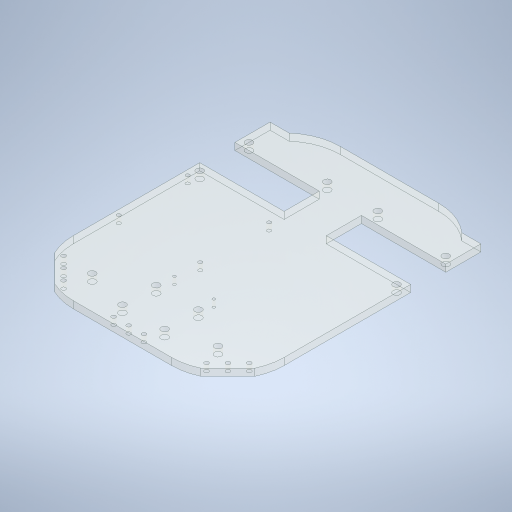
# Autodesk Inventor part: BaseP
Saved by Autodesk Inventor 2024 (Build 280153020, 153B)
## iProperties
Created: 2023-05-25
Part Number: BaseP
Material: Genérico
Document SubType Name: Modeling
Designer: victo
Density: 1 g/cm^3
Appearance: Transparente
Author: victo
Autodesk Inventor part; units mm, degrees
ref_plane "YZ Plane" through (0, 0, 0) normal (1, 0, 0) x (0, 1, 0)
ref_plane "XZ Plane" through (0, 0, 0) normal (0, 1, 0) x (-1, 0, 0)
ref_plane "XY Plane" through (0, 0, 0) normal (0, 0, 1) x (1, 0, 0)
sketch "Esboço1" plane through (0, 0, 0) normal (0, 1, 0) x (-1, 0, 0)
  line L0 (0, 0) -> (0, -190)
  line L1 (0, -190) -> (150, -190)
  line L2 (150, -190) -> (150, 0)
  line L3 (150, 0) -> (0, 0)
  dimension "d0" = 190
  dimension "d1" = 150
  constraints: 8 end point, 2 perpendicular, 1 parallel, 1 vertical
  measures "d0" distance of L0.start L0.end
  measures "d1" distance of L0.end L1.end
extrude "Extrusão1" add sketch "Esboço1" along normal mid plane 5
fillet "Arredondamento1" radius 40 1 edges at (0, 0, 0)
fillet "Arredondamento2" radius 40 3 edges at (-150, 0, 0) (0, 0, -190) (-150, 0, -190)
sketch "Esboço2" plane through (0, 2.5, 0) normal (0, 1, 0) x (1, 0, 0)
  line L0 (-110, 0) -> (-40, 0) projected
  line L1 (-150, 150) -> (-150, 40) projected
  line L2 (0, 40) -> (0, 150) projected
  line L3 (0, 110) -> (5, 110)
  line L4 (-150, 110) -> (-155, 110)
  line L5 (-155, 110) -> (-155, 175)
  line L6 (-155, 175) -> (-150, 175)
  line L7 (0, 175) -> (5, 175)
  line L8 (5, 175) -> (5, 110)
  line L9 (-155, 175) -> (-155, 180)
  line L10 (-155, 180) -> (-115.1221, 180)
  line L11 (-155, 110) -> (-155, 105)
  line L12 (-155, 105) -> (-150, 105)
  line L13 (5, 110) -> (5, 105)
  line L14 (5, 105) -> (0, 105)
  line L15 (-115.1221, 180) -> (-136.4575, 180)
  arc A0 (-110, 190) -> (-150, 150) centre (-110, 150) ccw projected
  line L16 (5, 175) -> (5, 180)
  line L17 (5, 180) -> (11.9999, 180)
  line L18 (-150, 175) -> (-141.225, 175)
  line L19 (0, 175) -> (-8.775, 175)
  arc A1 (0, 150) -> (-40, 190) centre (-40, 150) ccw projected
  line L20 (11.9999, 180) -> (-13.5425, 180)
  line L21 (0, 150) -> (0, 175)
  arc A2 (-110, 190) -> (-150, 150) centre (-110, 150) ccw projected
  line L22 (-150, 150) -> (-150, 175)
  point P0 (0, 0)
  point P1 (-136.4575, 180)
  dimension "d162" = 5
  dimension "d163" = 5
  dimension "d165" = 5
  dimension "d166" = 5
  constraints: 40 end point, 10 point on line, 7 perpendicular, 4 horizontal, 4 point on circle, 3 tangent, 2 vertical, 1 parallel
  measures "d162" distance of L3.start L3.end
  measures "d163" distance of L4.start L4.end
  measures "d165" distance of L5.end L9.end
  measures "d166" distance of L4.end L11.end
sketch "Esboço5" plane through (0, 2.5, 0) normal (0, 1, 0) x (1, 0, 0)
  circle A0 centre (-120.0001, 23.5) radius 2.5
  circle A1 centre (-30.5501, 23.5) radius 2.5
  circle A2 centre (-92.8994, 163.5564) radius 2.5
  circle A3 centre (-56.8994, 163.5564) radius 2.5
  point P0 (0, 0)
  dimension "d69" = 5
  dimension "d70" = 5
  dimension "d116" = 5
  dimension "d117" = 5
  constraints: 4 centre point
  measures "d69" diameter of A0
  measures "d70" diameter of A1
  measures "d116" diameter of A2
  measures "d117" diameter of A3
extrude "Extrusão17" cut sketch "Esboço5" against normal through all
extrude "Extrusão20" add sketch "Esboço2" against normal blind 5 contours L22 L18 A0 | L1 L12 L11 L4 | L18 L6 L9 L10 A0 | L2 L3 L13 L14 | A1 L19 L21 | A1 L20 L16 L7 L19
sketch "Esboço7" plane through (0, 2.5, 0) normal (0, 1, 0) x (1, 0, 0)
  line L0 (-150, 110) -> (-150, 175) projected
  line L1 (-126.8835, 155.0003) -> (-150, 155.0003)
  line L2 (-28.2595, 155.0003) -> (0, 155.0003)
  line L3 (-126.8835, 130.0003) -> (-150, 130.0003)
  line L4 (-126.8835, 130.0003) -> (-90, 130.0003)
  line L5 (-90, 130.0003) -> (-90, 155.0003)
  line L6 (-90, 155.0003) -> (-126.8835, 155.0003)
  line L7 (-28.2595, 130.0003) -> (0, 130.0003)
  line L8 (0, 175) -> (0, 110) projected
  line L9 (-28.2595, 130.0003) -> (-60, 130.0003)
  line L10 (-60, 130.0003) -> (-60, 155.0003)
  line L11 (-60, 155.0003) -> (-28.2595, 155.0003)
  line L12 (0, 155.0003) -> (0, 130.0003)
  line L13 (-150, 155.0003) -> (-150, 130.0003)
  point P0 (0, 0)
  point P1 (0, 142.5003)
  point P2 (-150, 142.5)
  point P3 (-90, 142.5003)
  dimension "d170" = 25
  dimension "d216" = 60
  dimension "d252" = 60
  constraints: 24 end point, 7 perpendicular, 7 point on line, 3 midpoint, 1 collinear, 1 horizontal
  measures "d170" distance of L3.start L1.start
  measures "d216" distance from line of point (0, 142.5) L10
  measures "d252" distance of point (-150, 142.5) point (-90, 142.5)
sketch "Esboço8" plane through (0, 2.5, 0) normal (0, 1, 0) x (1, 0, 0)
  line L0 (0, 175) -> (0, 110) projected
  circle A0 centre (-5, 125.0003) radius 2.5
  line L1 (-150, 155.0003) -> (-84.9995, 155.0003) projected
  circle A1 centre (-145.0006, 160.0003) radius 2.5
  circle A2 centre (-145, 125.0003) radius 2.5
  circle A3 centre (-5, 160.0003) radius 2.5
  point P0 (0, 0)
  point P1 (0, 130.0003)
  dimension "d180" = 5
  dimension "d186" = 5
  dimension "d187" = 5
  dimension "d264" = 5
  constraints: 4 centre point
  measures "d180" diameter of A0
  measures "d186" diameter of A1
  measures "d187" diameter of A2
  measures "d264" diameter of A3
extrude "Extrusão30" cut sketch "Esboço7" against normal through all
extrude "Extrusão32" cut sketch "Esboço8" against normal through all
sketch "Esboço10" plane through (0, 2.5, 0) normal (0, 1, 0) x (1, 0, 0)
  line L0 (5, 180) -> (-13.5425, 180) projected
  line L1 (0, 180) -> (0, 104.8979)
  line L2 (0, 104.8979) -> (5, 104.8979)
  line L3 (5, 104.8979) -> (5, 180)
  line L4 (5, 180) -> (0, 180)
  line L5 (-150, 175) -> (-150, 155.0003) projected
  line L6 (-150, 175) -> (-150, 180)
  line L7 (-136.4575, 180) -> (-155, 180) projected
  line L8 (-150, 180) -> (-155, 180)
  line L9 (-155, 180) -> (-155, 104.8979)
  line L10 (-155, 104.8979) -> (-150, 104.8979)
  line L11 (-150, 175) -> (-150, 104.8979)
  point P0 (0, 0)
  constraints: 18 end point, 5 perpendicular, 5 point on line, 2 collinear, 1 vertical
extrude "Extrusão33" cut sketch "Esboço10" against normal through all
sketch "Esboço6" plane through (0, 2.5, 0) normal (0, 1, 0) x (1, 0, 0)
  line L0 (-40, 0) -> (-110, 0) projected
  line L1 (-75, 0) -> (-57.5, 0)
  line L2 (-92.5, 45) -> (-92.5, 0)
  line L3 (-75, 0) -> (-92.5, 0)
  line L4 (-92.5, 45) -> (-57.5, 45)
  line L5 (-58.75, 54.5) -> (-58.75, 42.5)
  circle A0 centre (-69.65, 48.6) radius 2.5
  line L6 (-75, 45) -> (-86, 45)
  line L7 (-86, 45) -> (-86, 57)
  line L8 (-86, 57) -> (-64, 57)
  line L9 (-64, 57) -> (-64, 45)
  circle A1 centre (-89.0185, 51) radius 1
  circle A2 centre (-60.9815, 51) radius 1
  line L10 (-60, 39) -> (-90, 39)
  line L11 (-60, 15) -> (-90, 15)
  circle A3 centre (-90, 39) radius 2.5
  circle A4 centre (-60, 39) radius 2.5
  circle A5 centre (-60, 15) radius 2.5
  circle A6 centre (-90, 15) radius 2.5
  point P0 (0, 0)
  dimension "d137" = 45
  dimension "d138" = 35
  dimension "d159" = 5
  dimension "d206" = 11
  dimension "d207" = 12
  dimension "d208" = 22
  dimension "d210" = 2
  dimension "d211" = 2
  dimension "d349" = 5
  dimension "d350" = 5
  dimension "d351" = 5
  dimension "d352" = 5
  constraints: 22 end point, 7 centre point, 4 coincident, 4 perpendicular, 4 point on line, 2 midpoint, 1 collinear, 1 horizontal
  measures "d137" distance of L1.end L4.end
  measures "d138" distance of L4.end L2.start
  measures "d159" diameter of A0
  measures "d206" distance of L6.start L6.end
  measures "d207" distance of L6.end L7.end
  measures "d208" distance of L7.end L8.end
  measures "d210" diameter of A1
  measures "d211" diameter of A2
  measures "d349" diameter of A3
  measures "d350" diameter of A4
  measures "d351" diameter of A5
  measures "d352" diameter of A6
sketch "Esboço11" plane through (0, 2.5, 0) normal (0, 1, 0) x (1, 0, 0)
  line L0 (-150, 130.0003) -> (-150, 40) projected
  circle A0 centre (-146.5001, 117.8649) radius 1.375
  circle A1 centre (-88.5001, 117.8649) radius 1.375
  circle A2 centre (-88.5001, 68.8649) radius 1.375
  circle A3 centre (-146.5001, 68.8649) radius 1.375
  point P0 (0, 0)
  dimension "d292" = 2.75
  dimension "d293" = 2.75
  dimension "d294" = 2.75
  dimension "d295" = 2.75
  constraints: 4 centre point
  measures "d292" diameter of A0
  measures "d293" diameter of A1
  measures "d294" diameter of A2
  measures "d295" diameter of A3
extrude "Extrusão35" cut sketch "Esboço11" against normal through all
extrude "Extrusão39" cut sketch "Esboço6" against normal through all contours A1 | A2 | A3 | A4 | A5 | A6
sketch "Esboço13" plane through (0, 2.5, 0) normal (0, 1, 0) x (1, 0, 0)
  circle A0 centre (-142.1978, 23.0054) radius 1.5 projected
  arc A1 (-150, 40) -> (-110, 0) centre (-110, 40) ccw projected
  circle A2 centre (-126.995, 7.8026) radius 1.5 projected
  line L0 (-146.2103, 23.0054) -> (-126.995, 3.7899)
  line L1 (-146.2103, 23.0054) -> (-146.2103, 3.7899)
  line L2 (-146.2103, 3.7899) -> (-126.995, 3.7899)
  circle A3 centre (-7.8022, 23.0054) radius 1.5 projected
  arc A4 (-40, 0) -> (0, 40) centre (-40, 40) ccw projected
  circle A5 centre (-23.005, 7.8026) radius 1.5 projected
  line L3 (-3.7897, 23.0054) -> (-23.005, 3.7899)
  line L4 (-3.7897, 23.0054) -> (-3.7897, 3.7899)
  line L5 (-3.7897, 3.7899) -> (-23.005, 3.7899)
  point P0 (0, 0)
  constraints: 12 end point, 3 point on circle, 2 perpendicular, 2 vertical, 1 point on line
extrude "Extrusão41" cut sketch "Esboço13" against normal through all contours L0 A1 | A1 L2 L1 | L3 A4 | A4 L4 L5
sketch "Esboço12" plane through (0, 2.5, 0) normal (0, 1, 0) x (1, 0, 0)
  line L0 (-40, 0) -> (-110, 0) projected
  line L1 (-53.5, 10) -> (-53.5, 17)
  line L2 (-53.5, 17) -> (-96.5, 17)
  line L3 (-96.5, 17) -> (-96.5, 10)
  arc A0 (-40, 0) -> (0, 40) centre (-40, 40) ccw projected
  arc A1 (-150, 40) -> (-110, 0) centre (-110, 40) ccw projected
  line L4 (-110, 0) -> (-150, 40)
  line L5 (-150, 40) -> (-145.0503, 44.9497)
  line L6 (-145.0503, 44.9497) -> (-105.0503, 4.9497)
  line L7 (-40, 0) -> (0, 40)
  line L8 (0, 40) -> (-4.9497, 44.9497)
  line L9 (-4.9497, 44.9497) -> (-44.9497, 4.9497)
  line L10 (-44.9497, 4.9497) -> (-40, 0)
  line L11 (-110, 0) -> (-105.0503, 4.9497)
  line L12 (-112.3225, 2.3225) -> (-109.1405, 5.5045)
  circle A2 centre (-85.75, 4.5) radius 1.5
  circle A3 centre (-75, 4.5) radius 1.5
  circle A4 centre (-64.25, 4.5) radius 1.5
  line L13 (-134.4196, 30.7835) -> (-137.6016, 27.6016)
  line L14 (-126.8182, 23.1821) -> (-130, 20)
  line L15 (-119.2168, 15.5807) -> (-122.3988, 12.3988)
  line L16 (-30.7832, 15.5807) -> (-27.6012, 12.3988)
  line L17 (-23.1818, 23.1821) -> (-19.9998, 20.0002)
  line L18 (-15.5804, 30.7835) -> (-12.3984, 27.6016)
  line L19 (-146.2103, 23.0054) -> (-126.995, 3.7899) projected
  circle A5 centre (-125.819, 8.9785) radius 1.5
  circle A6 centre (-133.4203, 16.5797) radius 1.5
  circle A7 centre (-141.0218, 24.1813) radius 1.5
  line L20 (-3.7897, 23.0054) -> (-23.005, 3.7899) projected
  circle A8 centre (-24.181, 8.9785) radius 1.5
  circle A9 centre (-16.5796, 16.5799) radius 1.5
  circle A10 centre (-8.9782, 24.1813) radius 1.5
  point P0 (0, 0)
  dimension "d301" = 7
  dimension "d310" = 7
  dimension "d311" = 7
  dimension "d325" = 4.5
  dimension "d356" = 3
  dimension "d357" = 3
  dimension "d358" = 3
  dimension "d374" = 3
  dimension "d375" = 3
  dimension "d376" = 3
  dimension "d379" = 3
  dimension "d380" = 3
  dimension "d381" = 3
  constraints: 36 end point, 12 perpendicular, 9 centre point, 6 point on line, 1 midpoint, 1 point on circle, 1 vertical
  measures "d301" distance of L1.start L1.end
  measures "d310" distance of L4.end L5.end
  measures "d311" distance of L7.end L8.end
  measures "d325" distance of L12.start L12.end
  measures "d356" diameter of A2
  measures "d357" diameter of A3
  measures "d358" diameter of A4
  measures "d374" diameter of A5
  measures "d375" diameter of A6
  measures "d376" diameter of A7
  measures "d379" diameter of A8
  measures "d380" diameter of A9
  measures "d381" diameter of A10
extrude "Extrusão42" cut sketch "Esboço12" against normal through all contours A2 | A3 | A4 | A5 | A6 | A7 | A8 | A9 | A10
